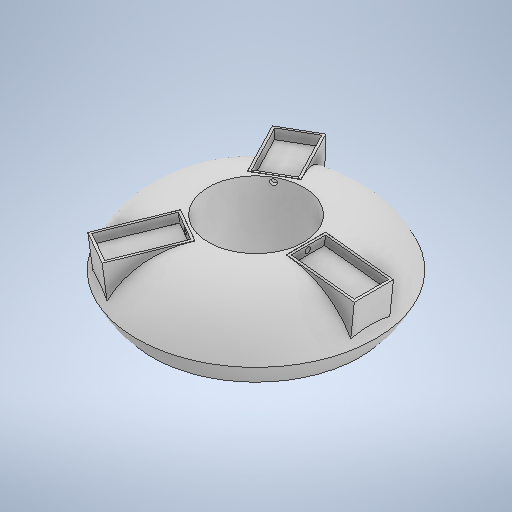
# Autodesk Inventor part: Water Sensor Bouy
Saved by Autodesk Inventor 2025 (Build 290162000, 162)
## iProperties
Created: 2024-06-17
Part Number: Water Sensor Bouy
Material: Generic
Document SubType Name: Modeling
Designer: track
Density: 1 g/cm^3
Appearance: Default
Author: track
## iProperties of the stored document Water Sensor Bouy_3DPrint.ipt
Created: 2024-06-17
Part Number: Water Sensor Bouy_3DPrint
Material: Generic
Document SubType Name: Modeling
Designer: track
Density: 1 g/cm^3
Appearance: Default
Author: track
Autodesk Inventor part; units mm, degrees
ref_plane "YZ Plane" through (0, 0, 0) normal (1, 0, 0) x (0, 1, 0)
ref_plane "XZ Plane" through (0, 0, 0) normal (0, 1, 0) x (-1, 0, 0)
ref_plane "XY Plane" through (0, 0, 0) normal (0, 0, 1) x (1, 0, 0)
sketch "Sketch1" plane through (0, 0, 0) normal (0, 0, 1) x (1, 0, 0)
  line L0 (0, 0) -> (0, 76.2)
  line L1 (50.7, 0) -> (50.7, 101.6)
  line L2 (50.7, 50.8) -> (126.9, 50.8)
  arc A0 (126.9, 50.8) -> (50.7, 101.6) centre (50.7, 19.05) ccw
  arc A1 (50.7, 0) -> (126.9, 50.8) centre (50.7, 82.55) ccw
  line L3 (50.7, 25.4) -> (110.2683, 25.4)
  line L4 (60.7, 90.9075) -> (60.7, 10.6925)
  arc A2 (60.7, 10.6925) -> (115.9337, 50.8) centre (50.7, 82.55) ccw
  arc A3 (115.9337, 50.8) -> (60.7, 90.9075) centre (50.7, 19.05) ccw
  line L5 (60.7, 31.75) -> (102.4964, 31.75)
  point P0 (60.7, 50.8)
  point P1 (60.7, 25.4)
  dimension "d0" = 101.6
  dimension "d1" = 50.7
  dimension "d2" = 50.8
  dimension "d3" = 0
  dimension "d4" = 76.2
  dimension "d24" = 82.55
  dimension "d27" = 25.4
  dimension "d31" = 6.35
  dimension "d33" = 10
  constraints: 12 end point, 10 point on circle, 4 centre point, 4 point on line, 2 horizontal, 2 vertical, 1 midpoint, 1 parallel, 2 other
  measures "d0" distance of L1.start L1.end
  measures "d1" distance between parallel lines of L1 L0
  measures "d2" distance from line of L1.end L2
  measures "d3" vertical distance of L0.start L1.start
  measures "d4" distance of L2.start L2.end
  measures "d24" radius of A0
  measures "d27" distance from line of L1.start L3
  measures "d31" distance between parallel lines of L3 L5
  measures "d33" distance between parallel lines of L1 L4
revolve "Revolution1" add sketch "Sketch1" angle 360 about axis through (0, 0, 0) along (0, 1, 0) contours L1 L2 L4 L3 | L3 A2 L2 A1 | L1 A0 L2 A3 L4 | L4 L5 A2 L3
sketch "Sketch6" plane through (0, 0, 0) normal (0, 0, 1) x (1, 0, 0)
  arc A0 (126.9, 50.8) -> (50.7, 101.6) centre (50.7, 19.05) ccw projected
  line L0 (50.7, 101.6) -> (-50.7, 101.6) projected
  arc A1 (121.82, 60.96) -> (50.7, 101.6) centre (50.7, 19.05) ccw
  line L1 (59.5439, 101.1249) -> (46.0594, 50.8)
  line L2 (115.9337, 50.8) -> (-115.9337, 50.8) projected
  point P0 (0, 0)
  dimension "d34" = 75
  dimension "d35" = 12.7
  constraints: 4 point on circle, 2 end point, 1 centre point, 1 concentric, 1 point on line
  measures "d34" angle of L2 L1
  measures "d35" distance from line of A0.centre L1
ref_plane "Work Plane4" through (59.5439, 101.1249, 0) normal (0.1071338, 0.9942446, 0) x (-0.9942446, 0.1071338, 0)
sketch "Sketch7" plane through (59.5439, 101.1249, 0) normal (0.1071338, 0.9942446, 0) x (-0.9942446, 0.1071338, 0)
  line L0 (3.9173, 18.25) -> (-63.5827, 18.25)
  line L1 (-63.5827, 18.25) -> (-63.5827, -18.25)
  line L2 (-63.5827, -18.25) -> (3.9173, -18.25)
  line L3 (3.9173, -18.25) -> (3.9173, 18.25)
  point P0 (48.3673, 0)
  dimension "d36" = 44.45
  dimension "d37" = 36.5
  dimension "d38" = 67.5
  dimension "d39" = 18.25
  constraints: 8 end point, 2 parallel, 1 horizontal, 1 perpendicular
  measures "d36" distance from line of point (48.367, 0) L3
  measures "d37" distance of L2.end L0.start
  measures "d38" distance of L1.end L2.end
  measures "d39" distance from line of point (48.367, 0) L2
extrude "Extrusion2" cut sketch "Sketch7" against normal blind 10
sketch "Sketch8" plane through (59.5439, 101.1249, 0) normal (0.1071338, 0.9942446, 0) x (-0.9942446, 0.1071338, 0)
  line L0 (3.9173, 18.25) -> (3.9173, -18.25) projected
  line L1 (3.9173, 18.25) -> (3.9173, -18.25)
  line L2 (3.9173, -18.25) -> (-63.5827, -18.25)
  line L3 (3.9173, -18.25) -> (-63.5827, -18.25)
  line L4 (-63.5827, -18.25) -> (-63.5827, 18.25)
  line L5 (-63.5827, 18.25) -> (3.9173, 18.25)
  line L6 (6.4573, -20.79) -> (6.4573, 20.79)
  line L7 (6.4573, 20.79) -> (-66.1227, 20.79)
  line L8 (-66.1227, 20.79) -> (-66.1227, -20.79)
  line L9 (6.4573, -20.79) -> (-66.1227, -20.79)
  point P0 (48.3673, 0)
  dimension "d42" = 67.5
  dimension "d43" = 2.54
  dimension "d45" = 2.54
  constraints: 18 end point, 4 perpendicular, 1 collinear, 1 parallel, 2 other
  measures "d42" distance of L4.end L0.start
  measures "d43" distance between parallel lines of L2 L9
  measures "d45" distance between parallel lines of L7 L5
extrude "Extrusion3" add sketch "Sketch8" against normal up to surface
sketch "Sketch9" plane through (58.4726, 91.1824, 0) normal (0.1071338, 0.9942446, 0) x (0.9942446, -0.1071338, 0)
  line L0 (63.5827, 18.25) -> (63.5827, -18.25) projected
  line L1 (-3.9173, -18.25) -> (-3.9173, 18.25) projected
  line L2 (63.5827, -18.25) -> (-3.9173, -18.25)
  line L3 (-3.9173, -18.25) -> (-3.9173, 18.25)
  line L4 (-3.9173, 18.25) -> (63.5827, 18.25)
  line L5 (63.5827, 18.25) -> (63.5827, -18.25)
  point P0 (-48.3673, 0)
  point P1 (-3.9173, -18.25)
  point P2 (63.5827, 18.25)
  constraints: 8 end point, 2 parallel, 1 horizontal, 1 perpendicular
extrude "Extrusion4" add sketch "Sketch9" against normal blind 10
pattern_circular "Circular Pattern1" count 3 over 360 about axis through (0, 19.05, 0) along (0, 1, 0) of "Extrusion2", "Extrusion3", "Extrusion4"
sketch "Sketch11" plane through (0, 25.4, 0) normal (0, -1, 0) x (1, 0, 0)
  circle A0 centre (76.9897, -44.45) radius 3.81
  circle A1 centre (76.9897, -44.45) radius 3.81 projected
  point P0 (0, 0)
  constraints: 2 concentric, 1 centre point
extrude "Extrusion6" cut sketch "Sketch11" against normal blind 11
sketch "Sketch12" plane through (54.5778, 91.6021, 18.25) normal (0.9942446, -0.1071338, 0) x (0, 0, -1)
  circle A0 centre (18.25, 5) radius 3
  line L0 (0, 10) -> (36.5, 10) projected
  point P0 (18.25, -96.922)
  dimension "d63" = 5
  dimension "d64" = 6
  dimension "d65" = 18.25
  constraints: 1 centre point
  measures "d63" distance from line of L0 A0.centre
  measures "d64" diameter of A0
  measures "d65" horizontal distance of L0.end A0.centre
extrude "Extrusion7" cut sketch "Sketch12" against normal up to surface round surface about axis through (0, 63.5, 0) along (0, 1, 0) radius 50.7 far side no
pattern_circular "Circular Pattern2" count 3 over 360 about axis through (0, 63.5, 0) along (0, 1, 0) of "Extrusion7"
pattern_circular "Circular Pattern3" count 3 over 360 about axis through (0, 63.5, 0) along (0, 1, 0) of "Extrusion6"
body "Solid1"
